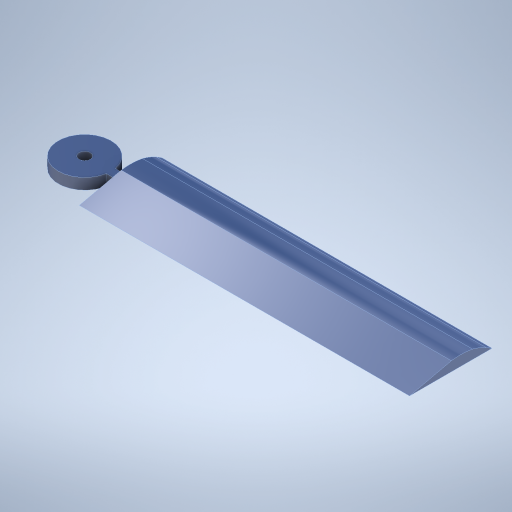
# Autodesk Inventor part: elevator
Saved by Autodesk Inventor 2023 (Build 270158000, 158)
## iProperties
Created: 2023-05-23
Part Number: elevator
Material: Generic
Document SubType Name: Modeling
Designer: Sujeet Kumar
Density: 1 g/cm^3
Appearance: Flaked Satin - Blue
Mass: 144.424 g
Surface Area: 521.082 cm^2
Volume: 144.424 cm^3
Author: Sujeet Kumar
Autodesk Inventor part; units mm, degrees
ref_plane "YZ Plane" through (0, 0, 0) normal (1, 0, 0) x (0, 1, 0)
ref_plane "XZ Plane" through (0, 0, 0) normal (0, 1, 0) x (-1, 0, 0)
ref_plane "XY Plane" through (0, 0, 0) normal (0, 0, 1) x (1, 0, 0)
sketch "Sketch1" plane through (0, 0, 0) normal (1, 0, 0) x (0, 1, 0)
  line L0 (0, 0) -> (0, -75)
  line L1 (0, -75) -> (3.365, -69.5807)
  line L2 (8.696, -38.0184) -> (0, 0)
  arc A0 (0, -75) -> (5.1288, -67.1329) centre (-33.3696, -47.6401) ccw
  arc A1 (0, -75) -> (8.2317, -57.2892) centre (-44.922, -43.3526) ccw
  arc A2 (8.2317, -57.2892) -> (8.696, -38.0184) centre (-47.0413, -46.3165) ccw
  point P0 (13.3125, -58.2014)
  dimension "d0" = 75
  constraints: 7 point on circle, 6 end point, 3 centre point, 1 point on line, 1 tangent, 1 vertical
  measures "d0" distance of L0.start L0.end
extrude "Extrusion1" add sketch "Sketch1" along normal blind 300 contours L2 A2 A1 L1 L0
sketch "Sketch2" plane through (0, 0, 0) normal (-1, 0, 0) x (0, 0, 1)
  line L0 (-99.8775, 0) -> (-66.8775, 0)
  line L1 (0, 0) -> (-75, 0) projected
  line L2 (-30.8596, 6.469) -> (-38.8596, 6.469)
  line L3 (-38.8596, 6.469) -> (-38.8596, 0.469)
  line L4 (-38.8596, 0.469) -> (-30.8596, 0.469)
  line L5 (-30.8596, 0.469) -> (-30.8596, 6.469)
  arc A0 (-87.3159, 9.7453) -> (-75, 0) centre (-67.8231, -28.7531) ccw projected
  line L6 (-75, 0) -> (-36, 0)
  dimension "d3" = 33
  dimension "d4" = 8
  dimension "d5" = 6
  dimension "d15" = 39
  constraints: 12 end point, 2 parallel, 2 point on line, 1 horizontal, 1 perpendicular, 1 other
  measures "d3" distance of L0.start L0.end
  measures "d4" distance of L4.end L3.end
  measures "d5" distance of L3.end L2.end
  measures "d15" distance of L1.end L6.end
extrude "Extrusion2" add sketch "Sketch2" along normal blind 30
sketch "Sketch3" plane through (0, 6.469, -56.2845) normal (0, 1, 0) x (1, 0, 0)
  line L0 (-30, -17.4249) -> (-30, -25.4249) projected
  circle A0 centre (-30, -21.4249) radius 24
  circle A1 centre (-30, -21.4249) radius 5.25
  point P0 (0, -56.2845)
  dimension "d8" = 48
  dimension "d9" = 10.5
  constraints: 2 centre point, 1 coincident, 1 midpoint
  measures "d8" diameter of A0
  measures "d9" diameter of A1
extrude "Extrusion3" add sketch "Sketch3" against normal blind 10
sketch "Sketch4" plane through (0, 6.469, -56.2845) normal (0, 1, 0) x (1, 0, 0)
  line L0 (-30, -17.4249) -> (-30, -25.4249) projected
  circle A0 centre (-30, -21.4249) radius 5.25
  point P0 (0, -56.2845)
  dimension "d12" = 10.5
  constraints: 1 centre point, 1 midpoint
  measures "d12" diameter of A0
extrude "Extrusion4" cut sketch "Sketch4" against normal blind 30
body "Solid1"
